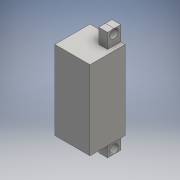
# Autodesk Inventor part: speaker
Saved by Autodesk Inventor 2016 (Build 200138000, 138)
## iProperties
Created: 2017-06-06
Part Number: speaker
Material: Generic
Document SubType Name: Modeling
Designer: fabio-note
Density: 1 g/cm^3
Appearance: Default
Author: fabio-note
Autodesk Inventor part; units mm, degrees
ref_plane "YZ Plane" through (0, 0, 0) normal (1, 0, 0) x (0, 1, 0)
ref_plane "XZ Plane" through (0, 0, 0) normal (0, 1, 0) x (-1, 0, 0)
ref_plane "XY Plane" through (0, 0, 0) normal (0, 0, 1) x (1, 0, 0)
sketch "Sketch1" plane through (0, 0, 0) normal (0, 1, 0) x (-1, 0, 0)
  line L0 (20, 45) -> (-20, 45)
  line L1 (-20, 45) -> (-20, -45)
  line L2 (-20, -45) -> (20, -45)
  line L3 (20, -45) -> (20, 45)
  point P0 (0, 0)
  point P1 (20, 0)
  point P2 (0, -45)
  dimension "d0" = 40
  dimension "d1" = 90
  constraints: 8 end point, 2 midpoint, 2 parallel, 1 horizontal, 1 horizontal alignment, 1 perpendicular, 1 vertical alignment
  measures "d0" distance between parallel lines of L1 L3
  measures "d1" distance between parallel lines of L2 L0
extrude "Extrusion1" add sketch "Sketch1" along normal blind 40
sketch "Sketch2" plane through (-20, 0, 45) normal (0, 0, 1) x (1, 0, 0)
  line L0 (0, 40) -> (40, 40) projected
  line L1 (35, 40) -> (25, 40)
  line L2 (25, 40) -> (25, 25)
  line L3 (25, 25) -> (35, 25)
  line L4 (35, 25) -> (35, 40)
  line L5 (40, 0) -> (40, 40) projected
  point P0 (20, 0)
  dimension "d4" = 5
  dimension "d5" = 10
  dimension "d6" = 15
  constraints: 8 end point, 2 parallel, 1 horizontal, 1 perpendicular, 1 point on line
  measures "d4" distance between parallel lines of L5 L4
  measures "d5" distance between parallel lines of L2 L4
  measures "d6" distance between parallel lines of L3 L0
extrude "Extrusion2" add sketch "Sketch2" along normal blind 17
sketch "Sketch3" plane through (15, 25, 45) normal (1, 0, 0) x (0, 0, -1)
  circle A0 centre (-12, 7.5) radius 5
  line L0 (-17, 0) -> (-17, 15) projected
  line L1 (0, 15) -> (-17, 15) projected
  point P0 (45, -25)
  dimension "d9" = 10
  dimension "d10" = 5
  dimension "d11" = 7.5
  constraints: 1 centre point
  measures "d9" diameter of A0
  measures "d10" distance from line of L0 A0.centre
  measures "d11" distance from line of L1 A0.centre
extrude "Extrusion3" cut sketch "Sketch3" against normal blind 17
mirror "Mirror3" about plane through (0, 0, 0) normal (0, 0, 1) of "Extrusion2", "Extrusion3"
sketch "Sketch4" plane through (0, 40, 0) normal (0, 1, 0) x (1, 0, 0)
  line L0 (-15, -40) -> (15, -40)
  line L1 (15, -40) -> (15, 40)
  line L2 (15, 40) -> (-15, 40)
  line L3 (-15, 40) -> (-15, -40)
  point P0 (0, 0)
  point P1 (-15, 0)
  point P2 (0, -40)
  dimension "d14" = 80
  dimension "d15" = 30
  constraints: 8 end point, 2 midpoint, 2 parallel, 1 horizontal, 1 horizontal alignment, 1 perpendicular, 1 vertical alignment
  measures "d14" distance between parallel lines of L2 L0
  measures "d15" distance between parallel lines of L1 L3
extrude "Extrusion4" cut sketch "Sketch4" against normal blind 2
body "Solid1"
